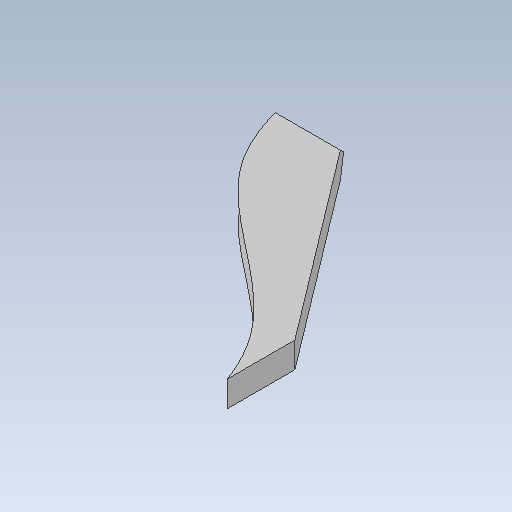
# Autodesk Inventor part: Secondary Beam
Saved by Autodesk Inventor 2021 (Build 250183000, 183)
## iProperties
Created: 2020-12-28
Part Number: Secondary Beam
Material: Generic
Document SubType Name: Modeling
Designer: Thomas Dodd
Density: 1 g/cm^3
Appearance: Default
Author: Thomas Dodd
Autodesk Inventor part; units mm, degrees
ref_plane "YZ Plane" through (0, 0, 0) normal (1, 0, 0) x (0, 1, 0)
ref_plane "XZ Plane" through (0, 0, 0) normal (0, 1, 0) x (-1, 0, 0)
ref_plane "XY Plane" through (0, 0, 0) normal (0, 0, 1) x (1, 0, 0)
sketch "Sketch1" plane through (0, 0, 0) normal (0, 1, 0) x (-1, 0, 0)
  spline S0 degree 4 poles (286, 0) (271, 60.691) (238, 121.382) (163, 182.0729) (80, 242.7639) (23, 303.4549) (0, 364.16) knots 1 1 1 1 1 2 3 4 4 4 4 4
  line L0 (0, 364.16) -> (0, 0) construction
  line L1 (0, 0) -> (286, 0) construction
  line L2 (0, 364.16) -> (0, 272.16)
  line L3 (286, 0) -> (206, 0)
  line L4 (206, 0) -> (0, 272.16)
  dimension "d0" = 286
  dimension "d1" = 364.16
  dimension "d2" = 92
  dimension "d3" = 80
  constraints: 10 end point, 2 point on line, 1 coincident, 1 perpendicular, 1 vertical, 3 other
  measures "d0" distance of L0.end L1.end
  measures "d1" distance of L0.start L0.end
  measures "d2" distance of L0.start L2.end
  measures "d3" distance of L1.end L3.end
extrude "Extrusion1" add sketch "Sketch1" along normal blind 35
sketch "Sketch2" plane through (0, 0, 364.16) normal (1, 0, 0) x (0, 0, -1)
  line L0 (364.16, 0) -> (364.16, 35) projected
  line L1 (364.16, 17.5) -> (346.66, 35)
  line L2 (364.16, 17.5) -> (388.9087, 17.5) construction
  line L3 (364.16, 17.5) -> (346.66, 0)
  line L4 (364.16, 17.5) -> (388.9087, 17.5) construction
  line L5 (92, 35) -> (364.16, 35) projected
  line L6 (92, 0) -> (364.16, 0) projected
  dimension "d9" = 135
  dimension "d10" = 135
  constraints: 8 end point, 2 equal length, 2 horizontal, 2 point on line, 1 midpoint
  measures "d9" angle of L2 L1
  measures "d10" angle of L3 L4
extrude "Extrusion2" cut sketch "Sketch2" against normal through all
sketch "Sketch3" plane through (0, 35, 0) normal (0, 1, 0) x (1, 0, 0)
  line L0 (-192.7541, -17.5) -> (-281.3669, -17.5) projected
  line L1 (0, -364.16) -> (0, -272.16) projected
  line L2 (0, -272.16) -> (-192.7541, -17.5) projected
  line L3 (-192.7541, -17.5) -> (-281.3669, -17.5) projected
  line L4 (-206, 0) -> (-192.7541, -17.5) projected
  line L5 (-206, 0) -> (-286, 0) projected
  point P0 (0, 0)
  constraints: 2 other
body "Solid1"
